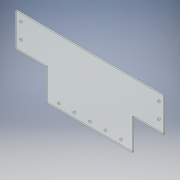
# Autodesk Inventor part: SUP_021_LexanShield
Saved by Autodesk Inventor 2018.3 (Build 223284000, 284)
## iProperties
Created: 2020-02-14
Part Number: SUP_021_LexanShield
Material: Generic
Document SubType Name: Modeling
Designer: 22barlalex
Density: 1 g/cm^3
Appearance: Clear
Author: 22barlalex
Autodesk Inventor part; units mm, degrees
ref_plane "YZ Plane" through (0, 0, 0) normal (1, 0, 0) x (0, 1, 0)
ref_plane "XZ Plane" through (0, 0, 0) normal (0, 1, 0) x (-1, 0, 0)
ref_plane "XY Plane" through (0, 0, 0) normal (0, 0, 1) x (1, 0, 0)
sketch "Sketch1" plane through (0, 0, 0) normal (0, 0, 1) x (1, 0, 0)
  line L0 (0, 0) -> (362.9152, 0)
  line L1 (362.9152, 0) -> (362.9152, 127)
  line L2 (362.9152, 127) -> (0, 127)
  line L3 (0, 127) -> (0, 0)
  dimension "d0" = 362.9152
  dimension "d1" = 127
  constraints: 8 end point, 2 parallel, 1 horizontal, 1 perpendicular
  measures "d0" distance of L2.end L1.end
  measures "d1" distance of L1.end L0.end
extrude "Extrusion1" add sketch "Sketch1" along normal blind 3.175
sketch "Sketch2" plane through (0, 0, 3.175) normal (0, 0, 1) x (1, 0, 0)
  line L0 (0, 127) -> (0, 0) projected
  line L1 (362.9152, 0) -> (362.9152, 127) projected
  line L2 (362.9152, 127) -> (0, 127) projected
  line L3 (0, 0) -> (362.9152, 0) projected
  point P0 (12.7, 25.4)
  point P1 (12.7, 63.5)
  point P2 (350.2152, 25.4)
  point P3 (350.2152, 63.5)
  point P4 (12.7, 101.6)
  point P5 (350.2152, 101.6)
  dimension "d4" = 12.7
  dimension "d5" = 12.7
  dimension "d6" = 12.7
  dimension "d7" = 12.7
  dimension "d8" = 12.7
  dimension "d9" = 12.7
  dimension "d10" = 25.4
  dimension "d11" = 25.4
  dimension "d12" = 38.1
  constraints: 3 horizontal alignment
  measures "d4" distance from line of L0 point (12.7, 25.4)
  measures "d5" distance from line of L0 point (12.7, 63.5)
  measures "d6" distance from line of L1 point (350.215, 25.4)
  measures "d7" distance from line of L1 point (350.215, 63.5)
  measures "d8" distance from line of L0 point (12.7, 101.6)
  measures "d9" distance from line of L1 point (350.215, 101.6)
  measures "d10" distance from line of L2 point (12.7, 101.6)
  measures "d11" distance from line of L3 point (12.7, 25.4)
  measures "d12" distance of point (12.7, 25.4) point (12.7, 63.5)
hole "Hole1" at (12.7, 25.4, 3.175) at (12.7, 63.5, 3.175) at (350.2152, 25.4, 3.175) at (350.2152, 63.5, 3.175) at (12.7, 101.6, 3.175) at (350.2152, 101.6, 3.175) direction (0, 0, -1) diameter 4.8514 end through all
sketch "Sketch3" plane through (0, 0, 3.175) normal (0, 0, 1) x (1, 0, 0)
  line L0 (0, 127) -> (0, 0) projected
  line L1 (362.9152, 0) -> (362.9152, 127) projected
  line L2 (0, 127) -> (362.9152, 127)
  line L3 (362.9152, 127) -> (362.9152, 82.55)
  line L4 (362.9152, 82.55) -> (0, 82.55)
  line L5 (0, 82.55) -> (0, 127)
  line L6 (0, 0) -> (362.9152, 0) projected
  line L7 (91.1104, 0) -> (300.3978, 0)
  line L8 (300.3978, 0) -> (300.3978, -76.2)
  line L9 (300.3978, -76.2) -> (91.1104, -76.2)
  line L10 (91.1104, -76.2) -> (91.1104, 0)
  dimension "d20" = 76.2
  dimension "d21" = 44.45
  constraints: 16 end point, 4 parallel, 2 horizontal, 2 perpendicular, 2 point on line
  measures "d20" distance between parallel lines of L6 L9
  measures "d21" distance between parallel lines of L4 L2
extrude "Extrusion2" cut sketch "Sketch3" against normal blind 25.4 contours L2 L1 L4 L0
sketch "Sketch4" plane through (0, 0, 3.175) normal (0, 0, 1) x (1, 0, 0)
  line L0 (0, 0) -> (362.9152, 0) projected
  line L1 (76.2, 0) -> (286.7152, 0)
  line L2 (286.7152, 0) -> (286.7152, -76.2)
  line L3 (286.7152, -76.2) -> (76.2, -76.2)
  line L4 (76.2, -76.2) -> (76.2, 0)
  line L5 (0, 82.55) -> (0, 0) projected
  line L6 (362.9152, 0) -> (362.9152, 82.55) projected
  dimension "d24" = 76.2
  dimension "d25" = 76.2
  dimension "d26" = 76.2
  constraints: 8 end point, 2 parallel, 1 horizontal, 1 perpendicular, 1 point on line
  measures "d24" distance of L1.end L2.end
  measures "d25" distance between parallel lines of L5 L4
  measures "d26" distance between parallel lines of L6 L2
extrude "Extrusion3" add sketch "Sketch4" against normal blind 3.175
sketch "Sketch5" plane through (0, 0, 3.175) normal (0, 0, 1) x (1, 0, 0)
  line L0 (286.7152, -76.2) -> (76.2, -76.2) projected
  line L1 (76.2, -76.2) -> (76.2, 0) projected
  point P0 (0, 0)
  point P1 (105.2576, -63.5)
  point P2 (143.3576, -63.5)
  point P3 (181.4576, -63.5)
  point P4 (219.5576, -63.5)
  point P5 (257.6576, -63.5)
  dimension "d29" = 38.1
  dimension "d30" = 38.1
  dimension "d31" = 38.1
  dimension "d32" = 38.1
  dimension "d33" = 12.7
  dimension "d34" = 29.0576
  constraints: 4 horizontal alignment
  measures "d29" distance of point (143.358, -63.5) point (105.258, -63.5)
  measures "d30" distance of point (181.458, -63.5) point (143.358, -63.5)
  measures "d31" distance of point (219.558, -63.5) point (181.458, -63.5)
  measures "d32" distance of point (257.658, -63.5) point (219.558, -63.5)
  measures "d33" distance from line of L0 point (105.258, -63.5)
  measures "d34" distance from line of L1 point (105.258, -63.5)
hole "Hole2" at (105.2576, -63.5, 3.175) at (143.3576, -63.5, 3.175) at (181.4576, -63.5, 3.175) at (219.5576, -63.5, 3.175) at (257.6576, -63.5, 3.175) direction (0, 0, -1) diameter 4.8514 end through all
body "Solid1"
